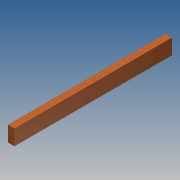
# Autodesk Inventor part: hubjig_side1
Saved by Autodesk Inventor 2014 SP1 (Build 180222100, 222)
## iProperties
Created: 2014-08-29
Part Number: hubjig_side1
Material: Wood (Cherry)
Document SubType Name: Modeling
Designer: Dave
Mass: 2168.01 g
Surface Area: 2648.38 cm^2
Volume: 3441.28 cm^3
Density: 0.63 g/cm^3
Appearance: Cherry - Natural Low Gloss
Author: Dave
Autodesk Inventor part; units mm, degrees
ref_plane "YZ Plane" through (0, 0, 0) normal (1, 0, 0) x (0, 1, 0)
ref_plane "XZ Plane" through (0, 0, 0) normal (0, 1, 0) x (-1, 0, 0)
ref_plane "XY Plane" through (0, 0, 0) normal (0, 0, 1) x (1, 0, 0)
sketch "Sketch1" plane through (0, 0, 0) normal (0, 0, 1) x (1, 0, 0)
  line L0 (0, 0) -> (38.1, 0)
  line L1 (38.1, 0) -> (38.1, 88.9)
  line L2 (38.1, 88.9) -> (0, 88.9)
  line L3 (0, 88.9) -> (0, 0)
  dimension "d0" = 38.1
  dimension "d1" = 88.9
  constraints: 8 end point, 2 parallel, 1 horizontal, 1 perpendicular
  measures "d0" distance of L0.start L0.end
  measures "d1" distance of L2.end L0.start
extrude "Extrusion1" add sketch "Sketch1" along normal blind 914.4
sketch "Sketch3" plane through (0, 0, 914.4) normal (0, 0, 1) x (1, 0, 0)
  line L0 (38.1, 88.9) -> (0, 88.9) projected
  line L1 (0, 88.9) -> (0, 0) projected
  circle A0 centre (19.05, 69.85) radius 6.0135
  circle A1 centre (19.05, 19.05) radius 6.0135
  dimension "d21" = 19.05
  dimension "d24" = 50.8
  constraints: 2 centre point, 1 vertical, 2 other
  measures "d21" distance from line of L0 A0.centre
  measures "d24" distance of A0.centre A1.centre
hole "Hole2" at (19.05, 69.85, 914.4) at (19.05, 19.05, 914.4) direction (0, 0, -1) diameter 5.1054 depth 25.4 tip angle 118 clearance for "Flat Head Machine Screw (82)" size "#10" standard "Ansi Unified Screw Threads"
sketch "Sketch4" plane through (0, 0, 0) normal (0, 0, -1) x (-1, 0, 0)
  line L0 (-38.1, 88.9) -> (0, 88.9) projected
  line L1 (-38.1, 0) -> (-38.1, 88.9) projected
  circle A0 centre (-19.05, 69.85) radius 5.0036
  circle A1 centre (-19.05, 19.05) radius 5.0036
  dimension "d36" = 19.05
  dimension "d39" = 50.8
  constraints: 2 centre point, 1 vertical, 2 other
  measures "d36" distance from line of L0 A0.centre
  measures "d39" distance of A0.centre A1.centre
hole "Hole3" at (19.05, 69.85, 0) at (19.05, 19.05, 0) direction (0, 0, 1) diameter 5.1054 depth 25.4 tip angle 118 clearance for "Flat Head Machine Screw (82)" size "#10" standard "Ansi Unified Screw Threads"
sketch "Sketch5" plane through (0, 88.9, 0) normal (0, 1, 0) x (1, 0, 0)
  line L0 (0, 0) -> (0, -914.4) projected
  line L1 (38.1, 0) -> (38.1, -914.4) projected
  line L2 (0, -457.2) -> (38.1, -457.2) construction
  circle A0 centre (19.05, -431.8) radius 3.4999
  circle A1 centre (19.05, -482.6) radius 3.4999
  dimension "d51" = 25.4
  constraints: 2 centre point, 2 end point, 2 midpoint, 1 symmetric about line, 1 other
  measures "d51" distance from line of L2 A0.centre
hole "Hole4" at (19.05, 88.9, 482.6) at (19.05, 88.9, 431.8) direction (0, -1, 0) diameter 5.1054 depth 25.4 tip angle 118 clearance for "Flat Head Machine Screw (82)" size "#10" standard "Ansi Unified Screw Threads"
body "Solid1"
